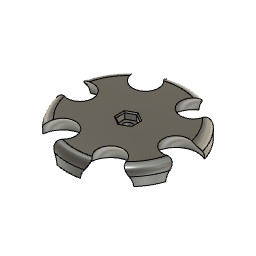
domekit_gheleguen_hub_x6_up_v2 (Autodesk Fusion 360 design; units mm, degrees)
Autodesk Fusion 360 part; units mm, degrees
sketch "Esquisse1" plane through (0, 0, 1) normal (0, 0, 1) x (1, 0, 0)
  circle A0 centre (0, 0) radius 27.75
  dimension "d1" = 55.5
  constraint coincident A0.centre origin
  measures "d1" diameter of A0
extrude "Extrusion1" add sketch "Esquisse1" along normal blind 7.5
ref_plane "Plan de construction3" through (0, 0, 0.5) normal (0, 0, -1) x (-1, 0, 0)
sketch "Esquisse2" plane through (0, 0, 0.5) normal (0, 0, -1) x (1, 0, 0)
  circle A0 centre (22, 0) radius 9.995
  circle A1 centre (0, 0) radius 27.75
  circle A2 centre (0, 0) radius 27.75
  dimension "d4" = 19.99
  dimension "d8" = 22
  measures "d4" diameter of A0
  measures "d8" distance of A1.centre A0.centre
sphere "SpherePrimitive1" cut diameter 19.9 placed x (1, 0, 0) y (0, -1, 0) z (0, 0, -1) at (22, 0, 0.5)
pattern_circular "Réseau C1" count 6 over 360 about axis through (0, 0, 1.75) along (0, 0, 1) of "SpherePrimitive1"
fillet "Congé1" chord length 5 6 edges at (24.0322, -13.875, 8.5) (24.0322, 13.875, 8.5) (0, 27.75, 8.5) (-24.0322, 13.875, 8.5) (-24.0322, -13.875, 8.5) (0, -27.75, 8.5)
hole "Perçage1" at (0, 0, 0.5) direction (0, 0, 1) diameter 4.3 depth 13 tip angle 180
sketch "Esquisse4" plane through (0, 0, 8.5) normal (0, 0, 1) x (-1, 0, 0)
  circle A0 centre (0, 0) radius 2.15
  spline S0 degree 3 poles (-6.8159, 23.2354) (-6.4153, 23.3529) (-6.0116, 23.4601) (-3.7717, 23.9931) (-1.8858, 24.2145) (0, 24.2145) (1.8858, 24.2145) (3.7717, 23.9931) (6.0116, 23.4601) (6.4153, 23.3529) (6.8159, 23.2354) knots -1.821842 -1.821842 -1.821842 -1.821842 -1.696594 -1.696594 -1.131062 -1.131062 -1.131062 -0.565531 -0.565531 -0.440283 -0.440283 -0.440283 -0.440283
  arc A1 (-16.7145, 17.5205) -> (-6.8159, 23.2354) centre (-11, 19.0526) ccw
  spline S1 degree 3 poles (-23.5304, 5.7149) (-23.4319, 6.1206) (-23.3228, 6.5239) (-22.6645, 8.7302) (-21.9132, 10.4741) (-20.9703, 12.1072) (-20.0275, 13.7404) (-18.8928, 15.2629) (-17.3113, 16.9362) (-17.0165, 17.2323) (-16.7145, 17.5205) knots -1.821842 -1.821842 -1.821842 -1.821842 -1.696594 -1.696594 -1.131062 -1.131062 -1.131062 -0.565531 -0.565531 -0.440283 -0.440283 -0.440283 -0.440283
  arc A2 (-23.5304, -5.7149) -> (-23.5304, 5.7149) centre (-22, 0) ccw
  spline S2 degree 3 poles (-16.7145, -17.5205) (-17.0165, -17.2323) (-17.3113, -16.9362) (-18.8928, -15.2629) (-20.0275, -13.7404) (-20.9703, -12.1072) (-21.9132, -10.4741) (-22.6645, -8.7302) (-23.3228, -6.5239) (-23.4319, -6.1206) (-23.5304, -5.7149) knots -1.821842 -1.821842 -1.821842 -1.821842 -1.696594 -1.696594 -1.131062 -1.131062 -1.131062 -0.565531 -0.565531 -0.440283 -0.440283 -0.440283 -0.440283
  arc A3 (-6.8159, -23.2354) -> (-16.7145, -17.5205) centre (-11, -19.0526) ccw
  spline S3 degree 3 poles (6.8159, -23.2354) (6.4153, -23.3529) (6.0116, -23.4601) (3.7717, -23.9931) (1.8858, -24.2145) (0, -24.2145) (-1.8858, -24.2145) (-3.7717, -23.9931) (-6.0116, -23.4601) (-6.4153, -23.3529) (-6.8159, -23.2354) knots -1.821842 -1.821842 -1.821842 -1.821842 -1.696594 -1.696594 -1.131062 -1.131062 -1.131062 -0.565531 -0.565531 -0.440283 -0.440283 -0.440283 -0.440283
  arc A4 (16.7145, -17.5205) -> (6.8159, -23.2354) centre (11, -19.0526) ccw
  spline S4 degree 3 poles (23.5304, -5.7149) (23.4319, -6.1206) (23.3228, -6.5239) (22.6645, -8.7302) (21.9132, -10.4741) (20.9703, -12.1072) (20.0275, -13.7404) (18.8928, -15.2629) (17.3113, -16.9362) (17.0165, -17.2323) (16.7145, -17.5205) knots -1.821842 -1.821842 -1.821842 -1.821842 -1.696594 -1.696594 -1.131062 -1.131062 -1.131062 -0.565531 -0.565531 -0.440283 -0.440283 -0.440283 -0.440283
  arc A5 (23.5304, 5.7149) -> (23.5304, -5.7149) centre (22, 0) ccw
  spline S5 degree 3 poles (16.7145, 17.5205) (17.0165, 17.2323) (17.3113, 16.9362) (18.8928, 15.2629) (20.0275, 13.7404) (20.9703, 12.1072) (21.9132, 10.4741) (22.6645, 8.7302) (23.3228, 6.5239) (23.4319, 6.1206) (23.5304, 5.7149) knots -1.821842 -1.821842 -1.821842 -1.821842 -1.696594 -1.696594 -1.131062 -1.131062 -1.131062 -0.565531 -0.565531 -0.440283 -0.440283 -0.440283 -0.440283
  arc A6 (6.8159, 23.2354) -> (16.7145, 17.5205) centre (11, 19.0526) ccw
  line L0 (-3.5024, -2.0165) -> (-0.0048, -4.0414)
  line L1 (-0.0048, -4.0414) -> (3.4976, -2.0249)
  line L2 (3.4976, -2.0249) -> (3.5024, 2.0165)
  line L3 (3.5024, 2.0165) -> (0.0048, 4.0414)
  line L4 (0.0048, 4.0414) -> (-3.4976, 2.0249)
  line L5 (-3.4976, 2.0249) -> (-3.5024, -2.0165)
  dimension "d24" = 3.5
  constraint coincident A0.centre origin
  measures "d24" distance of A0.centre L5
extrude "Extrusion2" cut sketch "Esquisse4" against normal blind 3 contours L0 L1 L2 L3 L4 L5
chamfer "Chanfrein1" distance 0.5 angle 45 6 edges at (-1.7464, 3.0332, 8.5) (1.7536, 3.029, 8.5) (3.5, -0.0042, 8.5) (1.7464, -3.0332, 8.5) (-1.7536, -3.029, 8.5) (-3.5, 0.0042, 8.5)
